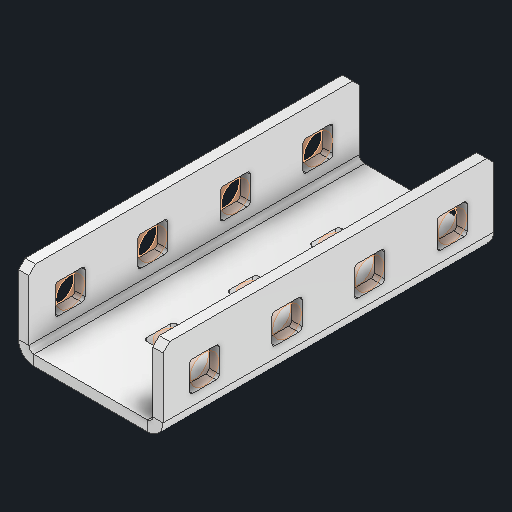
# Autodesk Inventor part: Alu C 1x2x1x35
Saved by Autodesk Inventor 2025 (Build 290162000, 162)
## iProperties
Created: 2022-07-28
Part Number: Alu C 1x2x1x35
Material: Generic
Document SubType Name: Sheet Metal
Designer: ylu12
Density: 1 g/cm^3
Sheet Metal Rule: Default
Appearance: Aluminum
Author: ylu12
Autodesk Inventor part; units mm, degrees
note: some values were not read from the file. Chosen so that the rebuilt part matches the saved one: hole positions of "Flange Pattern".
ref_plane "YZ Plane" through (0, 0, 0) normal (1, 0, 0) x (0, 1, 0)
ref_plane "XZ Plane" through (0, 0, 0) normal (0, 1, 0) x (-1, 0, 0)
sketch "Sketch1" plane through (0, 0, 0) normal (0, 1, 0) x (-1, 0, 0)
  line L0 (-11.1125, 0) -> (11.1125, 0)
  line L1 (11.1125, 0) -> (11.1125, -50.8)
  line L2 (11.1125, -50.8) -> (-11.1125, -50.8)
  line L3 (-11.1125, -50.8) -> (-11.1125, 0)
  line L4 (11.1125, 0) -> (-11.1125, -50.8) construction
  point P0 (0, 0)
  point P1 (0, 0)
  dimension "d0" = 22.225
  dimension "d1" = 50.8
  constraints: 10 end point, 2 parallel, 1 coincident, 1 horizontal, 1 midpoint, 1 perpendicular
  measures "d0" distance of L1.end L2.end
  measures "d1" distance of L0.end L1.end
extrude "Plate1" add sketch "Sketch1" along normal blind 1.5875
sketch "Sketch2" plane through (9.525, 0, -50.8) normal (1, 0, 0) x (0, 1, 0)
  line L0 (0, 50.8) -> (0, 0)
  line L1 (0, 0) -> (12.7, 0)
  line L2 (12.7, 0) -> (12.7, 50.8)
  line L3 (12.7, 50.8) -> (0, 50.8)
  constraints: 6 end point, 1 horizontal, 1 perpendicular, 1 vertical
edge flange "Flanges" height 12.7 angle 90 thickness 1.5875 bend radius 0.7937 thickness toward (1, 0, 0) relief tear relief width 1.5875 relief depth 0.7937 corner gap 1.5875 corner form 0 edges at (11.1125, 1.5875, -25.4) (-11.1125, 1.5875, -25.4) wall of the first edge with corners at (9.525, 0, 0) (9.525, 0, -50.8) (9.525, 12.7, -50.8) (9.525, 12.7, 0)
bend "Bend1"
corner "Corner1"
sketch "Sketch3" plane through (11.1125, 2.3812, -50.8) normal (1, 0, 0) x (0, 0, -1)
  line L0 (-46.2534, 6.2801) -> (-42.6466, 6.2801)
  line L1 (-42.1386, 5.7721) -> (-42.1386, 2.1653)
  line L2 (-42.6466, 1.6573) -> (-46.2534, 1.6573)
  line L3 (-46.7614, 2.1653) -> (-46.7614, 5.7721)
  arc A0 (-46.2534, 6.2801) -> (-46.7614, 5.7721) centre (-46.2534, 5.7721) ccw
  arc A1 (-42.1386, 5.7721) -> (-42.6466, 6.2801) centre (-42.6466, 5.7721) ccw
  arc A2 (-42.6466, 1.6573) -> (-42.1386, 2.1653) centre (-42.6466, 2.1653) ccw
  arc A3 (-46.7614, 2.1653) -> (-46.2534, 1.6573) centre (-46.2534, 2.1653) ccw
  line L4 (-50.8, 0) -> (-50.8, 10.3187) construction
  line L5 (-50.8, 10.3187) -> (0, 10.3187) construction
  line L6 (-46.2534, 5.7721) -> (-42.6466, 2.1653) construction
  point P0 (-50.8, -2.3813)
  point P1 (-42.1386, 1.6573)
  point P2 (-46.7614, 1.6573)
  point P3 (-44.45, 3.9687)
  dimension "d16" = 4.6228
  dimension "d17" = 0.508
  dimension "d20" = 6.35
  dimension "d21" = 6.35
  constraints: 10 end point, 8 point on circle, 8 tangent, 4 centre point, 4 point on line, 3 equal radius, 2 parallel, 2 perpendicular, 1 horizontal, 1 midpoint
  measures "d16" distance of point (-42.139, 1.657) point (-46.761, 1.657)
  measures "d17" radius of A0
  measures "d20" distance from line of point (-44.45, 3.969) L4
  measures "d21" distance from line of L5 point (-44.45, 3.969)
extrude "Flange Stamp" cut sketch "Sketch3" against normal blind 1.5875
sketch "Sketch7" plane through (11.1125, 2.3813, 0) normal (1, 0, 0) x (0, 0, -1)
  arc A0 (4.5466, 6.2802) -> (4.0386, 5.7722) centre (4.5466, 5.7722) ccw construction
  arc A1 (8.1534, 1.6573) -> (8.6614, 2.1653) centre (8.1534, 2.1653) ccw construction
  circle A2 centre (6.35, 3.9688) radius 2.1844
  line L0 (4.5466, 5.7722) -> (8.1534, 2.1653) construction
  point P0 (0, -2.3813)
  dimension "d46" = 4.3688
  constraints: 2 end point, 1 centre point, 1 midpoint
  measures "d46" diameter of A2
surface extrude "Flange Circle" sketch "Sketch7" against normal up to surface (1.5875 mm away) shown yes curves A2
ref_plane "Flange Pattern Plane" through (11.1125, 6.35, -4.5466) normal (0, 1, 0) x (1, 0, 0)
sketch "Flange Pattern Sketch" plane through (11.1125, 6.35, -4.5466) normal (0, 1, 0) x (1, 0, 0)
  line L0 (0, 3.6068) -> (0, 0) construction
  line L1 (-26.67, -4.5466) -> (4.445, -4.5466) construction
  line L2 (0, 0) -> (-1.5875, 0) construction
  point P0 (-11.1125, -4.5466)
  point P1 (0, 1.8034)
  point P2 (0, 14.5034)
  point P3 (0, 27.2034)
  point P4 (0, 39.9034)
  point P5 (-22.225, 1.8034)
  point P6 (-22.225, 14.5034)
  point P7 (-22.225, 27.2034)
  point P8 (-22.225, 39.9034)
  dimension "d40" = 12.7
  dimension "d121" = 22.225
  constraints: 1 horizontal, 1 midpoint, 1 vertical, 7 other
  measures "d40" distance of point (0, 1.803) point (0, 14.503)
  measures "d121" distance of point (0, 1.803) point (-22.225, 1.803)
pattern_sketch "Flange Pattern" of "Flange Circle", "Flange Stamp" from (11.1125, 6.35, -6.35) facing (1, 0, 0) copies at (11.1125, 6.35, -19.05) facing (1, 0, 0) at (11.1125, 6.35, -31.75) facing (1, 0, 0) at (11.1125, 6.35, -44.45) facing (1, 0, 0) at (-11.1125, 6.35, -6.35) facing (-1, 0, 0) at (-11.1125, 6.35, -19.05) facing (-1, 0, 0) at (-11.1125, 6.35, -31.75) facing (-1, 0, 0) at (-11.1125, 6.35, -44.45) facing (-1, 0, 0)
sketch "Sketch15" plane through (0, 0, 0) normal (0, -1, 0) x (1, 0, 0)
  line L0 (8.7312, 0) -> (-8.7312, 0) construction
  line L1 (1.8034, -10.3886) -> (-1.8034, -10.3886)
  line L2 (-2.3114, -10.8966) -> (-2.3114, -14.5034)
  line L3 (-1.8034, -15.0114) -> (1.8034, -15.0114)
  line L4 (2.3114, -14.5034) -> (2.3114, -10.8966)
  arc A0 (2.3114, -10.8966) -> (1.8034, -10.3886) centre (1.8034, -10.8966) ccw
  arc A1 (1.8034, -15.0114) -> (2.3114, -14.5034) centre (1.8034, -14.5034) ccw
  arc A2 (-1.8034, -10.3886) -> (-2.3114, -10.8966) centre (-1.8034, -10.8966) ccw
  arc A3 (-2.3114, -14.5034) -> (-1.8034, -15.0114) centre (-1.8034, -14.5034) ccw
  line L5 (1.8034, -10.8966) -> (-1.8034, -14.5034) construction
  line L6 (11.1125, 0) -> (11.1125, -50.8) construction
  line L7 (0, -12.7) -> (0, 0) construction
  point P0 (-2.3114, -15.0114)
  point P1 (2.3114, -15.0114)
  dimension "d106" = 4.6228
  dimension "d107" = 0.508
  dimension "d108" = 12.7
  constraints: 12 end point, 8 point on circle, 8 tangent, 4 centre point, 4 point on line, 3 equal radius, 2 parallel, 2 perpendicular, 1 horizontal, 1 midpoint, 1 vertical
  measures "d106" distance of point (2.311, -15.011) point (-2.311, -15.011)
  measures "d107" radius of A0
  measures "d108" distance from line of L0 L7.start
extrude "Center Stamp" cut sketch "Sketch15" against normal blind 1.5875
sketch "Sketch16" plane through (0, 0, 0) normal (0, -1, 0) x (1, 0, 0)
  circle A0 centre (0, -12.7) radius 2.1844
  line L0 (11.1125, 0) -> (11.1125, -50.8) construction
  arc A1 (-1.8034, -10.3886) -> (-2.3114, -10.8966) centre (-1.8034, -10.8966) ccw construction
  arc A2 (1.8034, -15.0114) -> (2.3114, -14.5034) centre (1.8034, -14.5034) ccw construction
  line L1 (-1.8034, -10.8966) -> (1.8034, -14.5034) construction
  point P0 (0, 0)
  dimension "d112" = 4.3688
  constraints: 2 end point, 1 centre point, 1 midpoint
  measures "d112" diameter of A0
surface extrude "Center Circle" sketch "Sketch16" against normal up to surface (1.5875 mm away) shown yes curves A0
pattern_linear "Center Pattern" count 3 spacing 12.7 along (0, 0, -1) of "Center Circle", "Center Stamp"
chamfer "End Chamfer" distance 1.016 angle 45 4 edges at (-10.3187, 12.7, -50.8) (10.3188, 12.7, -50.8) (-10.3187, 12.7, 0) (10.3187, 12.7, 0)
equation "\"d18\" = Thickness"
equation "\"d1\" = 12.7 * Length"
equation "\"d2\" = Thickness"
equation "\"d3\" = BendReliefWidth"
equation "\"d4\" = BendReliefDepth"
equation "\"d5\" = MinimumRemnant"
equation "\"d6\" = TransitionRadius"
equation "\"d10\" = CornerReliefSize"
equation "\"d11\" = GapSize"
equation "\"d12\" = JacobiRadiusSize"
equation "\"BendRadius\" = Thickness"
equation "\"BendReliefWidth\" = Thickness"
equation "\"BendReliefDepth\" = 0.5 * Thickness"
equation "\"CornerReliefSize\" = 4 * Thickness"
equation "\"MinimumRemnant\" = 2 * Thickness"
equation "\"TransitionRadius\" = BendRadius"
equation "\"JacobiRadiusSize\" = BendRadius"
equation "\"GapSize\" = Thickness"
equation "\"Thickness\" = 1.5875"
equation "\"Length\" = 4"
body "Solid1"
body "Srf1"
body "Srf2"
body "Srf786"
body "Srf823"
body "Srf824"
body "Srf825"
body "Srf826"
body "Srf827"
body "Srf828"
body "Srf889"
body "Srf890"
